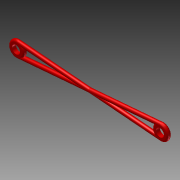
# Autodesk Inventor part: polycord cross proxy new
Saved by Autodesk Inventor 2011 SP1 (Build 150282100, 282)
## iProperties
Created: 2012-01-20
Part Number: polycord cross proxy new
Document SubType Name: Modeling
Designer: Christopher
Density: 1 g/cm^3
Author: Christopher
Autodesk Inventor part; units mm, degrees
ref_plane "YZ Plane" through (0, 0, 0) normal (1, 0, 0) x (0, 1, 0)
ref_plane "XZ Plane" through (0, 0, 0) normal (0, 1, 0) x (-1, 0, 0)
ref_plane "XY Plane" through (0, 0, 0) normal (0, 0, 1) x (1, 0, 0)
sketch "Sketch1" plane through (0, 0, 0) normal (0, 0, 1) x (1, 0, 0)
  circle A0 centre (172.8364, 23.614) radius 6.35
  circle A1 centre (-55.7636, 23.614) radius 6.35
  circle A2 centre (172.8364, 23.614) radius 12.7
  circle A3 centre (-55.7636, 23.614) radius 12.7
  line L0 (172.3072, 17.2861) -> (-54.7053, 36.2698)
  line L1 (-55.2344, 29.9419) -> (171.7781, 10.9582)
  line L2 (-55.2344, 17.2861) -> (171.7781, 36.2698)
  line L3 (172.3072, 29.9419) -> (-54.7053, 10.9582)
  line L4 (171.7781, 10.9582) -> (172.3072, 17.2861)
  line L5 (172.3072, 29.9419) -> (171.7781, 36.2698)
  line L6 (-54.7053, 10.9582) -> (-55.2344, 17.2861)
  line L7 (-55.2344, 29.9419) -> (-54.7053, 36.2698)
  line L8 (-55.2344, 17.2861) -> (-54.7053, 10.9582)
  point P0 (0, 0)
  dimension "d0" = 0
  dimension "d1" = 228.6
  dimension "d2" = 12.7
  dimension "d3" = 12.7
  dimension "d4" = 25.4
  dimension "d5" = 25.4
  constraints: 18 end point, 8 point on circle, 8 tangent, 4 centre point, 4 coincident, 1 collinear
  measures "d0" vertical distance of point (172.836, 23.614) point (-55.764, 23.614)
  measures "d1" distance of point (172.836, 23.614) point (-55.764, 23.614)
  measures "d2" diameter of A1
  measures "d3" diameter of A0
  measures "d4" diameter of A3
  measures "d5" diameter of A2
extrude "Extrusion1" add sketch "Sketch1" against normal blind 6.35 contours A0 L5 A2 L4 | A0 L0 A2 L3 | L3 A2 L5 | L4 A2 L0 | L3 L0 L2 A2 | A2 L1 L3 L0 | L3 L1 L2 L0 | L2 L1 A3 L0 | L3 A3 L2 L1 | L7 A1 L6 A3 | A3 L1 L7 | L6 L2 A3 | A3 L2 A1 L1
fillet "Fillet1" radius 3.175 24 edges at (1.9156, 31.535, 0) (-68.4636, 23.614, 0) (1.9156, 15.6931, 0) (1.9156, 31.535, -6.35) (-68.4636, 23.614, -6.35) (1.9156, 15.6931, -6.35) (115.1572, 31.535, -6.35) (185.5364, 23.614, -6.35) (115.1572, 15.6931, -6.35) (115.1572, 31.535, 0) (185.5364, 23.614, 0) (115.1572, 15.6931, 0) (128.9917, 20.9083, 0) (160.1364, 23.614, 0) (128.9917, 26.3197, 0) (-11.9189, 20.9083, 0) (-43.0636, 23.614, 0) (-11.9189, 26.3197, 0) (128.9917, 20.9083, -6.35) (128.9917, 26.3197, -6.35) (-11.9189, 20.9083, -6.35) (-11.9189, 26.3197, -6.35) (-43.0636, 23.614, -6.35) (160.1364, 23.614, -6.35)
body "Solid1"
